Autodesk Fusion 360 part; units mm, degrees
(part 2 of 2)
sketch "Board (2)" plane through (0, 0, 0) normal (0, 0, 1) x (1, 0, 0) in component "Board"
  line L0 (4.75, 0) -> (39.105, 0)
  arc A0 (0, 4.75) -> (4.75, 0) centre (4.75, 4.75) ccw
  line L1 (0, 27.9) -> (0, 4.75)
  line L2 (41.5, 27.94) -> (41.5, 32.002)
  arc A1 (39.105, 0) -> (43.855, 4.75) centre (39.105, 4.75) ccw
  arc A2 (41.5, 32.002) -> (39.105, 32.65) centre (39.105, 27.9) ccw
  line L3 (39.105, 32.65) -> (4.75, 32.65)
  arc A3 (4.75, 32.65) -> (0, 27.9) centre (4.75, 27.9) ccw
  line L4 (43.855, 4.75) -> (43.855, 27.94)
  line L5 (41.5, 27.94) -> (43.855, 27.94)
  arc A4 (1.6764, 7.5345) -> (1.6764, 8.8095) centre (1.6764, 8.172) ccw
  arc A5 (41.9, 18.0295) -> (41.9, 16.7545) centre (41.9, 17.392) ccw
  arc A6 (41.9, 16.7545) -> (41.9, 18.0295) centre (41.9, 17.392) ccw
  arc A7 (1.6764, 8.8095) -> (1.6764, 7.5345) centre (1.6764, 8.172) ccw
  arc A8 (1.6764, 8.8095) -> (1.6764, 7.5345) centre (1.6764, 8.172) ccw
  arc A9 (41.9, 18.0295) -> (41.9, 16.7545) centre (41.9, 17.392) ccw
  arc A10 (41.9, 16.7545) -> (41.9, 18.0295) centre (41.9, 17.392) ccw
  arc A11 (41.9, 18.0295) -> (41.9, 16.7545) centre (41.9, 17.392) ccw
  arc A12 (1.94, 29.0375) -> (1.94, 27.7625) centre (1.94, 28.4) ccw
  arc A13 (1.6764, 8.8095) -> (1.6764, 7.5345) centre (1.6764, 8.172) ccw
  arc A14 (1.6764, 7.5345) -> (1.6764, 8.8095) centre (1.6764, 8.172) ccw
  arc A15 (1.94, 27.7625) -> (1.94, 29.0375) centre (1.94, 28.4) ccw
  arc A16 (1.94, 29.0375) -> (1.94, 27.7625) centre (1.94, 28.4) ccw
  arc A17 (1.6764, 8.8095) -> (1.6764, 7.5345) centre (1.6764, 8.172) ccw
  arc A18 (1.94, 27.7625) -> (1.94, 29.0375) centre (1.94, 28.4) ccw
  arc A19 (41.9, 18.0295) -> (41.9, 16.7545) centre (41.9, 17.392) ccw
  arc A20 (41.9, 16.7545) -> (41.9, 18.0295) centre (41.9, 17.392) ccw
  arc A21 (41.9, 16.7545) -> (41.9, 18.0295) centre (41.9, 17.392) ccw
  arc A22 (1.6764, 7.5345) -> (1.6764, 8.8095) centre (1.6764, 8.172) ccw
  arc A23 (1.94, 29.0375) -> (1.94, 27.7625) centre (1.94, 28.4) ccw
  arc A24 (1.94, 27.7625) -> (1.94, 29.0375) centre (1.94, 28.4) ccw
  arc A25 (1.94, 27.7625) -> (1.94, 29.0375) centre (1.94, 28.4) ccw
  arc A26 (1.94, 29.0375) -> (1.94, 27.7625) centre (1.94, 28.4) ccw
  arc A27 (1.6764, 7.5345) -> (1.6764, 8.8095) centre (1.6764, 8.172) ccw
  arc A28 (1.94, 29.0692) -> (1.94, 27.7308) centre (1.94, 28.4) ccw
  arc A29 (1.6764, 8.8413) -> (1.6764, 7.5028) centre (1.6764, 8.172) ccw
  arc A30 (1.94, 27.7308) -> (1.94, 29.0692) centre (1.94, 28.4) ccw
  arc A31 (41.9, 18.0612) -> (41.9, 16.7228) centre (41.9, 17.392) ccw
  arc A32 (1.6764, 7.5028) -> (1.6764, 8.8413) centre (1.6764, 8.172) ccw
  arc A33 (41.9, 16.7228) -> (41.9, 18.0612) centre (41.9, 17.392) ccw
  arc A34 (1.94, 27.7308) -> (1.94, 29.0692) centre (1.94, 28.4) ccw
  arc A35 (41.9, 18.0612) -> (41.9, 16.7228) centre (41.9, 17.392) ccw
  arc A36 (1.6764, 8.8413) -> (1.6764, 7.5028) centre (1.6764, 8.172) ccw
  arc A37 (1.94, 29.0692) -> (1.94, 27.7308) centre (1.94, 28.4) ccw
  arc A38 (41.9, 16.7228) -> (41.9, 18.0612) centre (41.9, 17.392) ccw
  arc A39 (1.6764, 7.5028) -> (1.6764, 8.8413) centre (1.6764, 8.172) ccw
  point P0 (1.6764, 8.172)
  point P1 (41.9, 17.392)
  point P2 (1.94, 28.4)
extrude "Board" add sketch "Board (2)" along normal blind 3.1 separate body contours L0 A0 L1 L2 A1 A2 L3 A3 L4 L5 makes body 8 in component "Board"
move_body "Board (1)" bodies 8 to x (1, 0, 0) y (0, 1, 0) z (0, 0, 1) at (0, 0, 11.2) in component "Board"
sketch "Sketch1" plane through (0, 0, 0) normal (0, 0, 1) x (1, 0, 0) in component "Battery"
  line L0 (20, 15) -> (-20, 15)
  line L1 (-20, 15) -> (-20, -15)
  line L2 (-20, -15) -> (20, -15)
  line L3 (20, -15) -> (20, 15)
  line L4 (20, 15) -> (-20, -15) construction
  dimension "d443" = 40
  dimension "d444" = 30
  constraint horizontal L0
  constraint vertical L1
  constraint horizontal L2
  constraint vertical L3
  constraint midpoint L4 origin
  measures "d443" distance of L1 L3
  measures "d444" distance of L0 L2
extrude "Extrude1'" add sketch "Sketch1" along normal blind 11.2 separate body makes body 9 in component "Battery"
move_body "Align1'" bodies 9 to x (1, 0, 0) y (0, 1, 0) z (0, 0, 1) at (21.9275, 16.325, 0) in component "Battery"
component "Front" placed x (1, 0, 0) y (0, 1, 0) z (0, 0, 1) at (0, 0, 0)
component "Button" placed x (1, 0, 0) y (0, 1, 0) z (0, 0, 1) at (0, 0, 0)
component "Backplate" placed x (1, 0, 0) y (0, 1, 0) z (0, 0, 1) at (0, 0, 0)
component "Board" placed x (1, 0, 0) y (0, 1, 0) z (0, 0, 1) at (0, 0, 0)
component "Battery" placed x (1, 0, 0) y (0, 1, 0) z (0, 0, 1) at (0, 0, 0)
equation "BoardHeight = 32.65 mm"
equation "BoardWidth = 43.855 mm"
equation "EnclosureThickness = 1.5 mm"
equation "ImageSensorX = 33.5424 mm"
equation "ImageSensorY = 17.392 mm"
equation "MotionSensorX = 7.5 mm"
equation "MotionSensorY = 17.392 mm"
equation "MotionSensorDiameter = 9.3 mm + 0.5 mm + EnclosureMfgTol"
equation "LensProtrusionOutsideThickness = 13.5287 mm + 2 mm"
equation "LensProtrusionDepth = LensThreadDepth - MountPointDepth"
equation "OuterEdgeRadius = 6 mm"
equation "BoardRadius = 4.75 mm"
equation "MountPoint2X = 1.682 mm"
equation "MountPoint2Y = 8.172 mm"
equation "MountPointDepth = USBCReceptacleWidth + 0.3 mm"
equation "MountPoint3X = 41.9 mm"
equation "MountPoint3Y = 19 mm"
equation "MountPoint1X = 1.94 mm"
equation "MountPoint1Y = 28.4 mm"
equation "BackplateMountPointDepth = EnclosureDepth"
equation "BackplateMountPointWidth = 1.5 mm"
equation "HoleDiameter = 10 mm"
equation "BatteryWidth = 40 mm"
equation "BatteryHeight = 30 mm"
equation "BatteryThickness = 11 mm + 0.2 mm"
equation "BackplateOverlap = 0.2 mm"
equation "BackplateHoleOffset = ( BackplateMountPointWidth - EnclosureThickness ) / 2"
equation "ScrewHeadDiameter = 3 mm"
equation "ScrewHeadHeight = 1 mm"
equation "BackplateThickness = 1.5 mm"
equation "EnclosureDepth = FrontplateThickness + MountPointDepth + BoardThickness + BatteryThickness"
equation "BoardThickness = 3.1 mm"
equation "BoardEnclosureGap = 0.15 mm"
equation "USBCReceptacleCutoutWidth = USBCReceptacleWidth + USBCReceptacleTolerance + 2 * EnclosureMfgTol"
equation "USBCReceptacleCutoutHeight = USBCReceptacleHeight + USBCReceptacleTolerance + 2 * EnclosureMfgTol"
equation "USBCReceptacleCutoutRadius = 2.4 mm / 2 - 0.2 mm"
equation "USBCReceptacleY = 5.25348125 mm"
equation "USBCReceptacleWidth = 3.16 mm"
equation "d329 = BoardWidth"
equation "d330 = BoardHeight"
equation "d331 = BoardRadius"
equation "d332 = BoardEnclosureGap"
equation "d333 = EnclosureThickness"
equation "d334 = EnclosureDepth"
equation "d336 = BoardEnclosureGap + BackplateOverlap"
equation "d337 = BoardEnclosureGap + BackplateOverlap + BackplateGap"
equation "d350 = MotionSensorX"
equation "d351 = MotionSensorY"
equation "d352 = ImageSensorX"
equation "d353 = ImageSensorY"
equation "d354 = FrontplateThickness"
equation "d363 = MotionSensorDiameter"
equation "MountPointHeight = 3 mm"
equation "MountPointRadius = 1.5 mm"
equation "d443 = BatteryWidth"
equation "d444 = BatteryHeight"
equation "d445 = BatteryThickness"
equation "d492 = USBCReceptacleCutoutWidth"
equation "d493 = USBCReceptacleCutoutHeight"
equation "d497 = USBCReceptacleCutoutRadius"
equation "d498 = USBCReceptacleCutoutRadius"
equation "d499 = USBCReceptacleCutoutRadius"
equation "d502 = EnclosureMfgTol"
equation "d505 = -USBCReceptacleY"
equation "USBCReceptacleHeight = 8.94 mm"
equation "USBCReceptacleTolerance = 0.2 mm"
equation "EnclosureMfgTol = 0.1 mm"
equation "FrontplateThickness = 4.3 mm"
equation "LensThreadDepth = 9.2 mm" comment "Lens threaded region length + lens back focal length (BFL)"
equation "LensProtrusionInsideThickness = 13.0287 mm + 2 mm"
equation "d540 = -MountPointDepth"
equation "d542 = -MountPointDepth"
equation "d544 = LensProtrusionDepth"
equation "d546 = LensProtrusionDepth"
equation "d554 = LensProtrusionInsideThickness"
equation "d555 = LensProtrusionOutsideThickness"
equation "BackplateDovetailAngle = 10 deg"
equation "d575 = LensOringOutsideDiameter"
equation "LensOringOutsideDiameter = 13.5 mm + 0.1 mm"
equation "LensOringThickness = 1 mm"
equation "LensOringSeatDepth = 0.5 mm"
equation "d590 = MountPointDepth"
equation "d592 = MountPointDepth"
equation "d594 = LensProtrusionBoardGap"
equation "d596 = -MountPointDepth"
equation "LensProtrusionBoardGap = 0.25 mm" comment "Gap between inside lens protrusion and board"
equation "d598 = -MountPointDepth + LensProtrusionBoardGap"
equation "d599 = LensOringSeatDepth"
equation "d601 = -MountPointDepth"
equation "d602 = LensProtrusionBoardGap"
equation "d604 = MountPointHoleDepth"
equation "d611 = -MountPointDepth"
equation "MountPointHoleDepth = 5 mm"
equation "DovetailAngle = 10 deg"
equation "DovetailFillet = 0.5 mm"
equation "d641 = FrontplateFillet"
equation "FrontplateFillet = 2 mm"
equation "TextEngraveDepth = 0.25 mm"
equation "d647 = ImageSensorX"
equation "d648 = LEDY"
equation "d649 = FrontplateThickness"
equation "d650 = LEDHoleDiameter"
equation "LEDHoleDiameter = 0.75 mm"
equation "d653 = BoardThickness"
equation "d662 = MountPointHeight"
equation "d663 = MountPoint1Width"
equation "d664 = MountPoint2Width"
equation "d665 = MountPointHeight"
equation "d666 = MountPointHeight"
equation "d667 = MountPoint3Width"
equation "d668 = MountPoint2X"
equation "d669 = MountPoint2Y"
equation "d670 = MountPoint1X"
equation "d671 = MountPoint1Y"
equation "d672 = MountPoint3Y"
equation "d673 = MountPoint3X"
equation "BackplateIndentAngle = 10 deg"
equation "BackplateIndentOffset = 17 mm"
equation "BackplateGap = 0.075 mm"
equation "BackplateIndentRadius = 1 mm"
equation "BackplateIndentWidth = 5 mm"
equation "BackplateIndentHeight = 8 mm"
equation "BackplateIndentDepth = 0.5 mm"
equation "d762 = MountPointRadius"
equation "d763 = ButtonY"
equation "d764 = ImageSensorX"
equation "ButtonY = 4.75 mm"
equation "LEDY = 28.8 mm"
equation "ButtonDiameter = 3 mm"
equation "ButtonHoleDiameter = ButtonDiameter + ButtonEnclosureClearance"
equation "d771 = FrontplateThickness"
equation "d772 = ButtonHoleDiameter"
equation "d774 = ButtonDiameter"
equation "ButtonProtrusion = 0.6 mm"
equation "ButtonHeight = MountPointDepth + FrontplateThickness + ButtonProtrusion - TactileSwitchHeight"
equation "TactileSwitchHeight = 0.6 mm + 0.1 mm"
equation "d785 = ButtonHeight"
equation "d789 = ButtonProtrusion"
equation "d790 = ButtonHoleDiameter"
equation "ButtonStopperHeight = MountPointDepth - TactileSwitchHeight"
equation "ButtonStopperDiameter = 3.6 mm"
equation "ButtonEnclosureClearance = 0.2 mm"
equation "d794 = ButtonStopperDiameter"
equation "d795 = ButtonStopperHeight"
equation "BackplateMountPointHeight = 3 mm"
equation "d809 = BackplateMountPointY"
equation "BackplateMountPointY = BoardHeight / 2"
equation "d812 = BackplateMountPointWidth"
equation "d813 = MountPointHeight"
equation "d814 = BackplateMountPointY"
equation "d815 = BackplateMountPointDepth"
equation "d819 = BackplateMountPointWidth"
equation "d820 = MountPointHeight"
equation "d821 = BackplateMountPointY"
equation "d822 = MountPointHoleDepth"
equation "d825 = BackplateHoleOffset"
equation "d826 = BackplateHoleOffset"
equation "MountPoint1Width = 3 mm"
equation "MountPoint2Width = 3 mm"
equation "MountPoint3Width = 5 mm"
equation "d857 = EnclosureThickness"
equation "d858 = BackplateThickness"
equation "d860 = BackplateThickness"
equation "d862 = BackplateThickness"
equation "d872 = -TextEngraveDepth"
equation "d874 = BackplateEngravingRectWidth"
equation "d875 = BackplateEngravingRectHeight"
equation "d876 = BackplateEngravingRectRadius"
equation "BackplateEngravingRectRadius = 2.25 mm"
equation "BackplateEngravingRectWidth = 19 mm"
equation "BackplateEngravingRectHeight = 8 mm"
equation "d880 = -TextEngraveDepth"
equation "d882 = TextEngraveDepth"
named bodies: "Body", "Front", "USBCPlugCutout", "BackplateMountPoint1", "BackplateMountPoint2"
